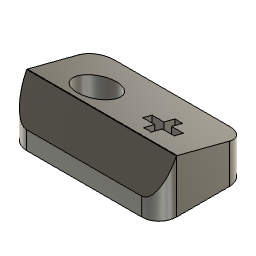
stab_adaptor (Autodesk Fusion 360 design; units mm, degrees)
Autodesk Fusion 360 part; units mm, degrees
sketch "Sketch1" plane through (0, 0, 0) normal (0, 0, 1) x (1, 0, 0)
  line L0 (0, 0) -> (21.55, 0)
  line L1 (21.55, 0) -> (21.55, 12.6)
  line L2 (21.55, 12.6) -> (0, 12.6)
  line L3 (0, 12.6) -> (0, 0)
  line L4 (0, 6.3) -> (21.55, 6.3) construction
  line L5 (6.3, 0) -> (6.3, 12.6) construction
  line L6 (0, 9.45) -> (6.3, 9.45) construction
  line L7 (3.15, 12.6) -> (3.15, 6.3) construction
  circle A0 centre (6.3, 6.3) radius 2.825
  line L8 (15.825, 12.6) -> (15.825, 0) construction
  line L9 (13.575, 5.635) -> (13.575, 6.965)
  line L10 (13.575, 6.965) -> (15.275, 6.965)
  line L11 (15.275, 6.965) -> (15.275, 8.55)
  line L12 (15.275, 8.55) -> (16.375, 8.55)
  line L13 (16.375, 8.55) -> (16.375, 6.965)
  line L14 (16.375, 6.965) -> (18.075, 6.965)
  line L15 (18.075, 6.965) -> (18.075, 5.635)
  line L16 (18.075, 5.635) -> (16.375, 5.635)
  line L17 (16.375, 5.635) -> (16.375, 4.05)
  line L18 (16.375, 4.05) -> (15.275, 4.05)
  line L19 (15.275, 4.05) -> (15.275, 5.635)
  line L20 (15.275, 5.635) -> (13.575, 5.635)
  line L21 (15.275, 5.635) -> (16.375, 6.965) construction
  line L22 (15.275, 6.965) -> (16.375, 5.635) construction
  line L23 (0, 6.3) -> (3.475, 6.3) construction
  line L24 (18.075, 6.3) -> (21.55, 6.3) construction
  dimension "d1" = 5.65
  dimension "d2" = 9.525
  dimension "d3" = 4.5
  dimension "d4" = 4.5
  dimension "d5" = 1.33
  dimension "d6" = 1.1
  dimension "d7" = 12.6
  constraint horizontal L0
  constraint vertical L1
  constraint horizontal L2
  constraint vertical L3
  constraint coincident L0.start L3.end
  constraint midpoint L3 L4.start
  constraint midpoint L1 L4.end
  constraint coincident L0 L5.start
  constraint coincident L2 L5.end
  constraint perpendicular L2 L5
  constraint coincident L3 L6.start
  constraint coincident L5 L6.end
  constraint perpendicular L5 L6
  constraint coincident L2 L7.start
  constraint coincident L4 L7.end
  constraint perpendicular L4 L7
  constraint equal L6 L7
  constraint midpoint L6 L7
  constraint midpoint L5 A0.centre
  constraint coincident L2 L8.start
  constraint coincident L0 L8.end
  constraint perpendicular L0 L8
  constraint perpendicular L4 L9
  constraint perpendicular L9 L10
  constraint perpendicular L4 L11
  constraint perpendicular L9 L12
  constraint perpendicular L12 L13
  constraint perpendicular L9 L14
  constraint perpendicular L12 L15
  constraint perpendicular L9 L16
  constraint perpendicular L12 L17
  constraint perpendicular L17 L18
  constraint perpendicular L18 L19
  constraint perpendicular L9 L20
  constraint midpoint L8 L21
  constraint midpoint L21 L22
  constraint equal L11 L19
  constraint equal L10 L14
  constraint equal L16 L20
  constraint equal L13 L17
  constraint coincident L4 L23.end
  constraint coincident A0 L23.end
  constraint midpoint L15 L24.start
  constraint perpendicular L1 L24
  constraint equal L23 L24
  measures "d1" diameter of A0
  measures "d2" distance of L5 L8
  measures "d3" distance of L9 L15
  measures "d4" distance of L12 L18
  measures "d5" distance of L14 L16
  measures "d6" distance of L11 L13
  measures "d7" distance of L0 L2
extrude "Extrude1" add sketch "Sketch1" along normal blind 7.6
chamfer "Chamfer1" distance 10 distance2 2.6 1 edges at (10.775, 12.6, 7.6) measured on face at (9.4929, 1.1819, 7.6)
chamfer "Chamfer2" distance 2.5 distance2 5 1 edges at (10.775, 0, 7.6) measured on face at (7.1833, 1.7333, 7.6)
fillet "Fillet2" radius 2.5 4 edges at (0, 12.6, 2.5) (0, 0, 1.3) (21.55, 0, 1.3) (21.55, 12.6, 2.5)
equation "d2 = ( 19.05 * Offset ) * 1 mm"
equation "d8 = Height"
equation "d13 = Height - 5 mm"
equation "Height = 7.6 mm"
equation "Offset = 0.5" comment "Offset distance in key units"
